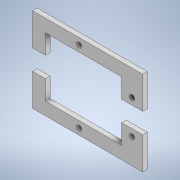
# Autodesk Inventor part: BASE_MID
Saved by Autodesk Inventor 2022 (Build 260153000, 153)
## iProperties
Created: 2022-11-15
Part Number: BASE_MID
Material: Genérico
Document SubType Name: Modeling
Designer: Usuario
Density: 1 g/cm^3
Appearance: Valor por defecto
Author: Usuario
Autodesk Inventor part; units mm, degrees
ref_plane "YZ Plane" through (0, 0, 0) normal (1, 0, 0) x (0, 1, 0)
ref_plane "XZ Plane" through (0, 0, 0) normal (0, 1, 0) x (-1, 0, 0)
ref_plane "XY Plane" through (0, 0, 0) normal (0, 0, 1) x (1, 0, 0)
sketch "Boceto1" plane through (0, 0, 0) normal (0, 0, 1) x (1, 0, 0)
  line L0 (-65, -50) -> (65, -50)
  line L1 (65, -50) -> (65, 50)
  line L2 (65, 50) -> (-65, 50)
  line L3 (-65, 50) -> (-65, -50)
  line L4 (-65, -50) -> (65, 50) construction
  line L5 (65, -50) -> (-65, 50) construction
  line L6 (-50, -35) -> (50, -35)
  line L7 (50, -35) -> (50, 35)
  line L8 (50, 35) -> (-50, 35)
  line L9 (-50, 35) -> (-50, -35)
  line L10 (-50, -35) -> (50, 35) construction
  line L11 (50, -35) -> (-50, 35) construction
  line L12 (0, 0) -> (-20, 0)
  line L13 (-20, 0) -> (-20, 35)
  line L14 (-50, 35) -> (50, 35)
  line L15 (-20, 0) -> (0, 0)
  line L16 (0, 0) -> (0, 35)
  line L17 (0, 35) -> (-20, 35)
  line L18 (-20, 35) -> (-20, 0)
  line L19 (50, -35) -> (-50, -35)
  line L20 (-20, 0) -> (0, 0)
  line L21 (0, 0) -> (0, -35)
  line L22 (0, -35) -> (-20, -35)
  line L23 (-20, -35) -> (-20, 0)
  line L24 (50, 35) -> (40, 35)
  line L25 (40, 35) -> (40, -35)
  line L26 (50, 35) -> (50, -35)
  line L27 (50, -35) -> (50, 35)
  line L28 (50, -35) -> (40, -35)
  line L29 (0, 0) -> (-20, 0)
  line L30 (-20, 35) -> (-20, -35)
  line L31 (-10, 0) -> (-10, 50)
  line L32 (65, 50) -> (-65, 50)
  line L33 (0, 35) -> (-10, 35)
  line L34 (-10, 35) -> (-10, 50)
  line L35 (-10, 50) -> (-10, 42.5)
  line L36 (-10, 0) -> (65, 0)
  line L37 (65, -50) -> (65, 50)
  line L38 (40, 35) -> (40, -35)
  line L39 (40, 0) -> (65, 0)
  line L40 (52.5, 0) -> (52.5, 20)
  circle A0 centre (-10, 42.5) radius 3
  circle A1 centre (52.5, 20) radius 3
  circle A2 centre (-10, -42.5) radius 3
  circle A3 centre (52.5, -20) radius 3
  line L41 (-50, 0) -> (-50, 12)
  line L42 (-50, 12) -> (-65, 12)
  line L43 (-65, 12) -> (-65, -12)
  line L44 (-65, -12) -> (-50, -12)
  line L45 (-50, 0) -> (-50, -12)
  line L46 (40, 0) -> (40, 12)
  line L47 (40, 12) -> (65, 12)
  line L48 (65, 12) -> (65, -12)
  line L49 (65, -12) -> (40, -12)
  point P0 (50, 12)
  point P1 (50, 18.3417)
  point P2 (52.5, 17)
  point P3 (52.5, 12)
  dimension "d0" = 130
  dimension "d2" = 100
  dimension "d4" = 20
  dimension "d7" = 6
  dimension "d9" = 12
  dimension "d10" = 24
  dimension "d11" = 12
  dimension "d12" = 24
  constraints: 100 end point, 13 midpoint, 13 perpendicular, 13 point on line, 8 parallel, 6 horizontal, 4 centre point, 2 coincident, 2 collinear, 2 symmetric about line, 2 vertical, 2 other
  measures "d0" distance of L2.end L1.end
  measures "d2" distance of L8.end L7.end
  measures "d4" distance of L12.start L12.end
  measures "d7" diameter of A0
  measures "d9" distance of L41.start L41.end
  measures "d10" distance of L42.end L43.end
  measures "d11" distance of L39.start L46.end
  measures "d12" distance of L47.end L48.end
extrude "Extrusión1" add sketch "Boceto1" along normal blind 5.5 contours L3 L44 L9 L6 L7 A3 L49 L1 L0 | L3 L2 L31 A0 L8 L9 L42 | L7 A3 L6 L25 L49 | L47 L40 A1 L7 L8 L31 A0 L2 L1 | L47 L7 A1 L40 | L47 L25 L8 L7 A1
